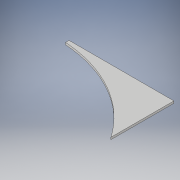
# Autodesk Inventor part: bottom-playfield
Saved by Autodesk Inventor 2017 (Build 210142000, 142)
## iProperties
Created: 2017-03-02
Part Number: bottom-playfield
Material: Generic
Document SubType Name: Modeling
Designer: John
Density: 1 g/cm^3
Appearance: Default
Author: John
Autodesk Inventor part; units mm, degrees
ref_plane "YZ Plane" through (0, 0, 0) normal (1, 0, 0) x (0, 1, 0)
ref_plane "XZ Plane" through (0, 0, 0) normal (0, 1, 0) x (-1, 0, 0)
ref_plane "XY Plane" through (0, 0, 0) normal (0, 0, 1) x (1, 0, 0)
sketch "Sketch1" plane through (0, 0, 0) normal (0, 1, 0) x (-1, 0, 0)
  line L0 (0, 90) -> (0, 0)
  line L1 (0, 0) -> (150, 0)
  line L2 (150, 0) -> (150, 5)
  line L3 (0, 90) -> (150, 5) construction
  arc A0 (0, 90) -> (150, 5) centre (163.9731, 204.5113) ccw
  point P0 (0, 0)
  dimension "d5" = 0
  dimension "d8" = 150
  dimension "d9" = 90
  dimension "d10" = 5
  dimension "d11" = 200
  constraints: 8 end point, 2 point on circle, 2 vertical, 1 centre point, 1 perpendicular
  measures "d5" distance of L0.end point (0, 0)
  measures "d8" distance of L0.end L1.end
  measures "d9" distance of L0.start L0.end
  measures "d10" distance of L1.end L2.end
  measures "d11" radius of A0
extrude "Extrusion1" add sketch "Sketch1" along normal blind 3
body "Solid1"
